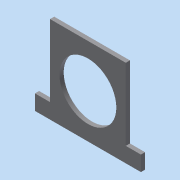
# Autodesk Inventor part: anillo2
Saved by Autodesk Inventor 2015 (Build 190159000, 159)
## iProperties
Created: 2017-09-29
Part Number: anillo2
Material: Generic
Document SubType Name: Modeling
Designer: macbook
Density: 1 g/cm^3
Appearance: Default
Author: macbook
Autodesk Inventor part; units mm, degrees
ref_plane "YZ Plane" through (0, 0, 0) normal (1, 0, 0) x (0, 1, 0)
ref_plane "XZ Plane" through (0, 0, 0) normal (0, 1, 0) x (-1, 0, 0)
ref_plane "XY Plane" through (0, 0, 0) normal (0, 0, 1) x (1, 0, 0)
sketch "Sketch1" plane through (0, 0, 0) normal (0, 0, 1) x (1, 0, 0)
  line L0 (100, 150) -> (0, 150)
  circle A0 centre (50, 207.5) radius 37.5
  line L1 (120, 170) -> (-20, 170)
  line L2 (0, 170) -> (100, 170)
  line L3 (100, 170) -> (100, 265)
  line L4 (100, 265) -> (0, 265)
  line L5 (0, 265) -> (0, 170)
  line L6 (-20, 170) -> (-20, 150)
  line L7 (-20, 150) -> (0, 150)
  line L8 (100, 150) -> (120, 150)
  line L9 (120, 150) -> (120, 170)
  point P0 (0, 0)
  dimension "d0" = 75
  dimension "d1" = 140
  dimension "d2" = 95
  constraints: 20 end point, 3 perpendicular, 2 parallel, 2 point on line, 1 centre point, 1 horizontal, 1 vertical
  measures "d0" diameter of A0
  measures "d1" distance of L1.end L1.start
  measures "d2" distance of L3.end L2.end
extrude "Extrusion1" add sketch "Sketch1" along normal blind 5.5
body "Solid1"
